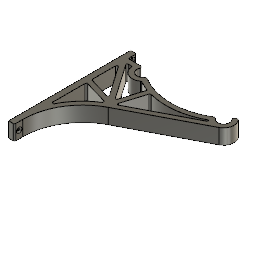
Shelf Bracket Filament (Autodesk Fusion 360 design; units mm, degrees)
Autodesk Fusion 360 part; units mm, degrees
ref_plane "WorkPlane1" through (-87.2, -39.4, 1) normal (0, -1, 0) x (1, 0, 0) in component "Filament Spool v1"
sketch "Sketch1" plane through (0, -39.4, 19) normal (0, -1, 0) x (1, 0, 0) in component "Filament Spool v1"
  line L0 (-70, -19) -> (-70, 13) construction
  line L1 (-81.2, -7.5) -> (-58.8, -7.5) construction
  circle A0 centre (-70, -7.5) radius 12.5 construction
  line L2 (-95.2, -19) -> (95.2, -19) construction
  line L3 (95.2, -19) -> (-95.2, -19) construction
  line L4 (0, -19) -> (0, -95.5696) construction
  line L5 (-70, -7.5) -> (0, -95.5696) construction
  circle A1 centre (0, -95.5696) radius 100
  circle A2 centre (0, -95.5696) radius 16
  circle A3 centre (0, -95.5696) radius 29
  dimension "d141" = 200
  dimension "d142" = 32
  dimension "d143" = 58
  measures "d141" diameter of A1
  measures "d142" diameter of A2
  measures "d143" diameter of A3
extrude "Extrude1" add sketch "Sketch1" against normal blind 31 contours A3 makes body 1 in component "Filament Spool v1"
extrude "Extrude2" add sketch "Sketch1" against normal blind 3 contours A1 bodies 1 in component "Filament Spool v1"
mirror "Mirror1" about plane through (0, -8.4, 19) normal (0, 1, 0) of bodies 1 makes body 2 in component "Filament Spool v1"
ref_plane "WorkPlane1" through (0, -35.4581, -18.5114) normal (0, 0, 1) x (1, 0, 0) in component "Bracket Hollow"
sketch "Shape" plane through (0, -35.4581, -18.5114) normal (0, 0, 1) x (1, 0, 0) in component "Bracket Hollow"
  circle A0 centre (0, 0) radius 100 construction
  circle A1 centre (0, 0) radius 16 construction
  circle A2 centre (-67.4303, -86.3069) radius 9.525 construction
  circle A3 centre (67.4303, -86.3069) radius 9.525 construction
  line L0 (0, 0) -> (0, -254.1299) construction
  line L1 (0, 0) -> (-67.4303, -86.3069) construction
  line L2 (0, 0) -> (67.4303, -86.3069) construction
  arc A4 (-79.6085, -70.7818) -> (83.1792, -66.5492) centre (0, 0) ccw construction
  arc A5 (-72.5254, -78.0234) -> (-58.1603, -89.2466) centre (-67.4303, -86.3069) ccw
  arc A6 (-85.1531, -86.0234) -> (-56.0327, -99.8815) centre (-67.4303, -86.3069) ccw
  arc A7 (58.1603, -89.2466) -> (72.5254, -78.0234) centre (67.4303, -86.3069) ccw
  arc A8 (56.0327, -99.8815) -> (78.2573, -72.2729) centre (67.4303, -86.3069) ccw
  arc A9 (-56.0327, -99.8815) -> (56.0327, -99.8815) centre (0, 0) ccw
  arc A10 (-58.1603, -89.2466) -> (58.1603, -89.2466) centre (0, 0) ccw
  arc A11 (72.5254, -78.0234) -> (78.2573, -72.2729) centre (0, 0) ccw
  line L3 (-85.1531, -86.0234) -> (-100, -86.0234)
  line L4 (-72.5254, -78.0234) -> (-100, -78.0234)
  line L5 (-100, -64.0234) -> (-110, -64.0234)
  line L6 (-110, -64.0234) -> (-110, -268.1299)
  line L7 (-110, -268.1299) -> (-100, -268.1299)
  line L8 (-100, -268.1299) -> (-100, -254.1299)
  line L9 (75.6148, -102.0291) -> (-46.1749, -165.4288)
  arc A12 (-46.1749, -165.4288) -> (-100, -254.1299) centre (0, -254.1299) ccw
  line L10 (67.4303, -86.3069) -> (75.6148, -102.0291) construction
  line L11 (-100, -254.1299) -> (0, -254.1299) construction
  line L12 (0, -254.1299) -> (-49.8689, -158.3328) construction
  line L13 (-49.8689, -158.3328) -> (58.7763, -101.7757)
  line L14 (-100, -64.0234) -> (-100, -268.1299) construction
  arc A13 (-49.8689, -158.3328) -> (-100, -213.3378) centre (0, -254.1299) ccw
  line L15 (-100, -78.0234) -> (-100, -64.0234)
  line L16 (-100, -86.0234) -> (-100, -213.3378)
  line L17 (-100, -86.0234) -> (-49.8689, -158.3328) construction
  line L18 (-95.1327, -86.0234) -> (-46.2923, -156.4709)
  line L19 (-100, -93.044) -> (-53.4023, -160.2566)
  line L20 (-49.8689, -158.3328) -> (0, 0) construction
  line L21 (-49.8689, -158.3328) -> (-100, -143.3378) construction
  line L22 (-51.232, -149.3459) -> (-38.1991, -107.9667)
  line L23 (-30.5687, -110.37) -> (-44.8527, -155.7215)
  line L24 (-54.7631, -161.0439) -> (-100, -147.5129)
  line L25 (-100, -139.1627) -> (-59.6614, -151.2286)
  line L26 (-100, -71.0234) -> (-110, -71.0234) construction
  line L27 (-100, -261.1299) -> (-110, -261.1299) construction
  line L28 (85.1553, -53.7492) -> (85.1553, -190) construction
  dimension "d28" = 19.05
  dimension "d29" = 19.05
  dimension "d33" = 8
  dimension "d36" = 38
  dimension "d37" = 3
  dimension "d38" = 0.2
  dimension "d39" = 8
  dimension "d41" = 0.2
  dimension "d42" = 8
  dimension "d44" = 8
  dimension "d46" = 10
  dimension "d47" = 8
  dimension "d49" = 14
  dimension "d50" = 62.5
  dimension "d51" = 8
  dimension "d52" = 8
  dimension "d53" = 8
  dimension "d54" = 70
  dimension "d60" = 14
  dimension "d61" = 204.8421
  measures "d28" diameter of A2
  measures "d29" diameter of A3
  measures "d33" distance of A9 A10
  measures "d36" angle of L0 L1
  measures "d38" distance of A2 A5
  measures "d39" distance of A5 A6
  measures "d41" distance of A3 A7
  measures "d42" distance of A7 A8
  measures "d47" distance of L3 L4
  measures "d50" angle of L11 L12
  measures "d51" distance of L18 L19
  measures "d52" distance of L24 L25
  measures "d53" distance of L22 L23
  measures "d61" distance of L5 L7
extrude "Extrude1'" add sketch "Shape" along normal mid plane 25.4 separate body contours A5 A7 A8 A10 A11 L4 L5 L6 L7 L8 L9 A12 L15 | L3 L13 A13 L16 L18 L19 | A9 L13 L18 L22 L23 | A13 L16 L19 L24 L25 makes body 3 in component "Bracket Hollow"
fillet "Fillet3" radius 2 18 edges at (-100, -99.4815, -18.5114) (-100, -113.4815, -18.5114) (-95.1327, -121.4815, -18.5114) (-100, -128.5021, -18.5114) (-100, -174.6208, -18.5114) (-100, -182.971, -18.5114) (-100, -248.7959, -18.5114) (-44.8527, -191.1796, -18.5114) (-51.232, -184.804, -18.5114) (-59.6614, -186.6867, -18.5114) (-54.7631, -196.5021, -18.5114) (58.7763, -137.2338, -18.5114) (56.0327, -135.3396, -18.5114) (-30.5687, -145.8281, -18.5114) (-38.1991, -143.4248, -18.5114) (-100, -303.5881, -18.5114) (-56.0327, -135.3396, -18.5114) (-85.1531, -121.4815, -18.5114) on bodies 3 in component "Bracket Hollow"
fillet "Fillet4" radius 3 5 edges at (58.1603, -124.7047, -18.5114) (78.2573, -107.731, -18.5114) (72.5254, -113.4815, -18.5114) (-58.1603, -124.7047, -18.5114) (-72.5254, -113.4815, -18.5114) on bodies 3 in component "Bracket Hollow"
ref_plane "WorkPlane5" through (-110, -201.5348, -18.5114) normal (-1, 0, 0) x (0, -1, 0) in component "Bracket Hollow"
sketch "Screw Holes" plane through (-110, -201.5348, -18.5114) normal (-1, 0, 0) x (0, 1, 0) in component "Bracket Hollow"
  line L0 (-100.0533, -12.7) -> (-100.0533, 12.7) construction
  line L1 (-100.0533, 12.7) -> (-88.0533, 12.7) construction
  line L2 (-88.0533, 12.7) -> (-88.0533, -12.7) construction
  line L3 (-88.0533, -12.7) -> (-100.0533, -12.7) construction
  line L4 (90.0533, -12.7) -> (90.0533, 12.7) construction
  line L5 (90.0533, 12.7) -> (100.0533, 12.7) construction
  line L6 (100.0533, 12.7) -> (100.0533, -12.7) construction
  line L7 (100.0533, -12.7) -> (90.0533, -12.7) construction
  line L8 (95.0533, -12.7) -> (95.0533, 12.7) construction
  line L9 (93.7353, -4.0672) -> (92.4173, -6.35)
  line L10 (92.4173, -6.35) -> (93.7353, -8.6328)
  line L11 (93.7353, -8.6328) -> (96.3712, -8.6328)
  line L12 (96.3712, -8.6328) -> (97.6892, -6.35)
  line L13 (97.6892, -6.35) -> (96.3712, -4.0672)
  line L14 (96.3712, -4.0672) -> (93.7353, -4.0672)
  line L15 (93.7353, 8.6328) -> (92.4173, 6.35)
  line L16 (92.4173, 6.35) -> (93.7353, 4.0672)
  line L17 (93.7353, 4.0672) -> (96.3712, 4.0672)
  line L18 (96.3712, 4.0672) -> (97.6892, 6.35)
  line L19 (97.6892, 6.35) -> (96.3712, 8.6328)
  line L20 (96.3712, 8.6328) -> (93.7353, 8.6328)
  line L21 (-94.0533, -12.7) -> (-94.0533, 12.7) construction
  line L22 (-92.7353, -2.2828) -> (-91.4173, 0)
  line L23 (-91.4173, 0) -> (-92.7353, 2.2828)
  line L24 (-92.7353, 2.2828) -> (-95.3712, 2.2828)
  line L25 (-95.3712, 2.2828) -> (-96.6892, 0)
  line L26 (-96.6892, 0) -> (-95.3712, -2.2828)
  line L27 (-95.3712, -2.2828) -> (-92.7353, -2.2828)
  line L28 (90.0533, 0) -> (100.0533, -12.7) construction
  line L29 (90.0533, 0) -> (100.0533, 12.7) construction
  dimension "d91" = 2.2828
  dimension "d92" = 2.2828
  dimension "d93" = 2.2828
  measures "d91" distance of L14
  measures "d92" distance of L20
  measures "d93" distance of origin L27
extrude "Extrude3" cut sketch "Screw Holes" against normal up to surface (10 mm away) bodies 3 in component "Bracket Hollow"
ref_plane "WorkPlane6" through (-110, -106.4815, -18.5114) normal (0, 1, 0) x (0, 0, -1) in component "Bracket Hollow"
sketch "Screw Bevel Top" plane through (-110, -106.4815, -18.5114) normal (0, 1, 0) x (1, 0, 0) in component "Bracket Hollow"
  line L0 (10, -8.6328) -> (10, -6.35) construction
  line L1 (10, -6.35) -> (10, -4.0672) construction
  line L2 (10, -4.0672) -> (10, -6.35) construction
  line L3 (10, -6.35) -> (10, -8.6328) construction
  line L4 (10, 4.0672) -> (10, 6.35) construction
  line L5 (10, 6.35) -> (10, 8.6328) construction
  line L6 (10, 8.6328) -> (10, 6.35) construction
  line L7 (10, 6.35) -> (10, 4.0672) construction
  line L8 (10, -12.7) -> (10, 12.7) construction
  line L9 (10, 12.7) -> (10, -12.7) construction
  line L10 (0, -6.35) -> (0, -8.6328) construction
  line L11 (0, -8.6328) -> (0, -6.35) construction
  line L12 (0, -6.35) -> (0, -4.0672) construction
  line L13 (0, -4.0672) -> (0, -6.35) construction
  line L14 (0, 6.35) -> (0, 4.0672) construction
  line L15 (0, 4.0672) -> (0, 6.35) construction
  line L16 (0, 6.35) -> (0, 8.6328) construction
  line L17 (0, 8.6328) -> (0, 6.35) construction
  line L18 (0, 0) -> (0, 2.2828) construction
  line L19 (0, 2.2828) -> (0, 0) construction
  line L20 (0, 0) -> (0, -2.2828) construction
  line L21 (0, -2.2828) -> (0, 0) construction
  line L22 (0, 12.7) -> (0, -12.7) construction
  line L23 (0, -12.7) -> (0, 12.7) construction
  line L24 (10, -6.35) -> (0, -6.35) construction
  line L25 (10, 6.35) -> (0, 6.35) construction
  line L26 (10, 1.9336) -> (4.8291, 6.35)
  line L27 (4.8291, 6.35) -> (10, 10.7664) construction
  line L28 (10, -10.7664) -> (4.8291, -6.35)
  line L29 (4.8291, -6.35) -> (10, -1.9336) construction
  line L30 (10, -10.7664) -> (10, -6.35)
  line L31 (10, -6.35) -> (4.8291, -6.35)
  line L32 (10, 1.9336) -> (10, 6.35)
  line L33 (10, 6.35) -> (4.8291, 6.35)
  dimension "d100" = 81
  dimension "d101" = 81
  dimension "d102" = 8.8328
  dimension "d103" = 8.8328
  measures "d100" angle of L26 L27
  measures "d101" angle of L28 L29
revolve "Revolve4" cut sketch "Screw Bevel Top" angle 360 about axis through (-100, -106.4815, -12.1614) along (-1, 0, 0) contours L28 L30 L31 bodies 3 in component "Bracket Hollow"
revolve "Revolve5" cut sketch "Screw Bevel Top" angle 360 about axis through (-100, -106.4815, -24.8614) along (-1, 0, 0) contours L26 L32 L33 bodies 3 in component "Bracket Hollow"
ref_plane "WorkPlane7" through (-110, -295.5881, -18.5114) normal (0, 1, 0) x (0, 0, -1) in component "Bracket Hollow"
sketch "Screw Bevel Bottom" plane through (-110, -295.5881, -18.5114) normal (0, 1, 0) x (1, 0, 0) in component "Bracket Hollow"
  line L0 (10, 2.2828) -> (10, 0) construction
  line L1 (10, 0) -> (10, -2.2828) construction
  line L2 (10, -2.2828) -> (10, 0) construction
  line L3 (10, 0) -> (10, 2.2828) construction
  line L4 (10, -12.7) -> (10, 12.7) construction
  line L5 (10, 12.7) -> (10, -12.7) construction
  line L6 (0, -6.35) -> (0, -8.6328) construction
  line L7 (0, -8.6328) -> (0, -6.35) construction
  line L8 (0, -6.35) -> (0, -4.0672) construction
  line L9 (0, -4.0672) -> (0, -6.35) construction
  line L10 (0, 6.35) -> (0, 4.0672) construction
  line L11 (0, 4.0672) -> (0, 6.35) construction
  line L12 (0, 6.35) -> (0, 8.6328) construction
  line L13 (0, 8.6328) -> (0, 6.35) construction
  line L14 (0, 0) -> (0, 2.2828) construction
  line L15 (0, 2.2828) -> (0, 0) construction
  line L16 (0, 0) -> (0, -2.2828) construction
  line L17 (0, -2.2828) -> (0, 0) construction
  line L18 (0, 12.7) -> (0, -12.7) construction
  line L19 (0, -12.7) -> (0, 12.7) construction
  line L20 (0, 0) -> (10, 0) construction
  line L21 (10, 4.4164) -> (4.8291, 0) construction
  line L22 (4.8291, 0) -> (10, -4.4164)
  line L23 (10, -4.4164) -> (10, 0)
  line L24 (10, 0) -> (4.8291, 0)
  dimension "d107" = 8.8328
  dimension "d108" = 81
  measures "d108" angle of L21 L22
revolve "Revolve6" cut sketch "Screw Bevel Bottom" angle 360 about axis through (-110, -295.5881, -18.5114) along (1, 0, 0) bodies 3 in component "Bracket Hollow"
ref_plane "WorkPlane1" through (0, -35.4581, -18.5114) normal (0, 0, 1) x (1, 0, 0) in component "Bracket Fill"
sketch "Shape (2)" plane through (0, -35.4581, -18.5114) normal (0, 0, 1) x (1, 0, 0) in component "Bracket Fill"
  circle A0 centre (0, 0) radius 100 construction
  circle A1 centre (0, 0) radius 16 construction
  circle A2 centre (-67.4303, -86.3069) radius 9.525 construction
  circle A3 centre (67.4303, -86.3069) radius 9.525 construction
  line L0 (0, 0) -> (0, -254.1299) construction
  line L1 (0, 0) -> (-67.4303, -86.3069) construction
  line L2 (0, 0) -> (67.4303, -86.3069) construction
  arc A4 (-79.6085, -70.7818) -> (83.1792, -66.5492) centre (0, 0) ccw construction
  arc A5 (-72.5254, -78.0234) -> (-58.1603, -89.2466) centre (-67.4303, -86.3069) ccw
  arc A6 (-85.1531, -86.0234) -> (-56.0327, -99.8815) centre (-67.4303, -86.3069) ccw
  arc A7 (58.1603, -89.2466) -> (72.5254, -78.0234) centre (67.4303, -86.3069) ccw
  arc A8 (56.0327, -99.8815) -> (78.2573, -72.2729) centre (67.4303, -86.3069) ccw
  arc A9 (-56.0327, -99.8815) -> (56.0327, -99.8815) centre (0, 0) ccw
  arc A10 (-58.1603, -89.2466) -> (58.1603, -89.2466) centre (0, 0) ccw
  arc A11 (72.5254, -78.0234) -> (78.2573, -72.2729) centre (0, 0) ccw
  line L3 (-85.1531, -86.0234) -> (-100, -86.0234)
  line L4 (-72.5254, -78.0234) -> (-100, -78.0234)
  line L5 (-100, -64.0234) -> (-110, -64.0234)
  line L6 (-110, -64.0234) -> (-110, -268.1299)
  line L7 (-110, -268.1299) -> (-100, -268.1299)
  line L8 (-100, -268.1299) -> (-100, -254.1299)
  line L9 (75.6148, -102.0291) -> (-46.1749, -165.4288)
  arc A12 (-46.1749, -165.4288) -> (-100, -254.1299) centre (0, -254.1299) ccw
  line L10 (67.4303, -86.3069) -> (75.6148, -102.0291) construction
  line L11 (-100, -254.1299) -> (0, -254.1299) construction
  line L12 (0, -254.1299) -> (-49.8689, -158.3328) construction
  line L13 (-49.8689, -158.3328) -> (58.7763, -101.7757)
  line L14 (-100, -64.0234) -> (-100, -268.1299) construction
  arc A13 (-49.8689, -158.3328) -> (-100, -213.3378) centre (0, -254.1299) ccw
  line L15 (-100, -78.0234) -> (-100, -64.0234)
  line L16 (-100, -86.0234) -> (-100, -213.3378)
  line L17 (-100, -86.0234) -> (-49.8689, -158.3328) construction
  line L18 (-95.1327, -86.0234) -> (-46.2923, -156.4709)
  line L19 (-100, -93.044) -> (-53.4023, -160.2566)
  line L20 (-49.8689, -158.3328) -> (0, 0) construction
  line L21 (-49.8689, -158.3328) -> (-100, -143.3378) construction
  line L22 (-51.232, -149.3459) -> (-38.1991, -107.9667)
  line L23 (-30.5687, -110.37) -> (-44.8527, -155.7215)
  line L24 (-54.7631, -161.0439) -> (-100, -147.5129)
  line L25 (-100, -139.1627) -> (-59.6614, -151.2286)
  line L26 (-100, -71.0234) -> (-110, -71.0234) construction
  line L27 (-100, -261.1299) -> (-110, -261.1299) construction
  line L28 (85.1553, -53.7492) -> (85.1553, -190) construction
  dimension "d28_1" = 19.05
  dimension "d29_1" = 19.05
  dimension "d33_1" = 8
  dimension "d36_1" = 38
  dimension "d37_1" = 3
  dimension "d38_1" = 0.2
  dimension "d39_1" = 8
  dimension "d41_1" = 0.2
  dimension "d42_1" = 8
  dimension "d44_1" = 8
  dimension "d46_1" = 10
  dimension "d47_1" = 8
  dimension "d49_1" = 14
  dimension "d50_1" = 62.5
  dimension "d51_1" = 8
  dimension "d52_1" = 8
  dimension "d53_1" = 8
  dimension "d54_1" = 70
  dimension "d60_1" = 14
  dimension "d61_1" = 204.8421
  measures "d28_1" diameter of A2
  measures "d29_1" diameter of A3
  measures "d33_1" distance of A9 A10
  measures "d36_1" angle of L0 L1
  measures "d38_1" distance of A2 A5
  measures "d39_1" distance of A5 A6
  measures "d41_1" distance of A3 A7
  measures "d42_1" distance of A7 A8
  measures "d47_1" distance of L3 L4
  measures "d50_1" angle of L11 L12
  measures "d51_1" distance of L18 L19
  measures "d52_1" distance of L24 L25
  measures "d53_1" distance of L22 L23
  measures "d61_1" distance of L5 L7
extrude "Extrude1''" add sketch "Shape (2)" along normal mid plane 25.4 separate body contours A5 A7 A8 A10 A11 L4 L5 L6 L7 L8 L9 A12 L15 | L3 L13 A13 L16 L18 L19 | A9 L13 L18 L22 L23 | A13 L16 L19 L24 L25 makes body 4 in component "Bracket Fill"
fillet "Fillet3'" radius 2 18 edges at (-100, -99.4815, -18.5114) (-100, -113.4815, -18.5114) (-95.1327, -121.4815, -18.5114) (-100, -128.5021, -18.5114) (-100, -174.6208, -18.5114) (-100, -182.971, -18.5114) (-100, -248.7959, -18.5114) (-44.8527, -191.1796, -18.5114) (-51.232, -184.804, -18.5114) (-59.6614, -186.6867, -18.5114) (-54.7631, -196.5021, -18.5114) (58.7763, -137.2338, -18.5114) (56.0327, -135.3396, -18.5114) (-30.5687, -145.8281, -18.5114) (-38.1991, -143.4248, -18.5114) (-100, -303.5881, -18.5114) (-56.0327, -135.3396, -18.5114) (-85.1531, -121.4815, -18.5114) on bodies 4 in component "Bracket Fill"
fillet "Fillet4'" radius 3 5 edges at (58.1603, -124.7047, -18.5114) (78.2573, -107.731, -18.5114) (72.5254, -113.4815, -18.5114) (-58.1603, -124.7047, -18.5114) (-72.5254, -113.4815, -18.5114) on bodies 4 in component "Bracket Fill"
ref_plane "WorkPlane5" through (-110, -201.5348, -18.5114) normal (-1, 0, 0) x (0, -1, 0) in component "Bracket Fill"
sketch "Screw Holes (2)" plane through (-110, -201.5348, -18.5114) normal (-1, 0, 0) x (0, 1, 0) in component "Bracket Fill"
  line L0 (-100.0533, -12.7) -> (-100.0533, 12.7) construction
  line L1 (-100.0533, 12.7) -> (-88.0533, 12.7) construction
  line L2 (-88.0533, 12.7) -> (-88.0533, -12.7) construction
  line L3 (-88.0533, -12.7) -> (-100.0533, -12.7) construction
  line L4 (90.0533, -12.7) -> (90.0533, 12.7) construction
  line L5 (90.0533, 12.7) -> (100.0533, 12.7) construction
  line L6 (100.0533, 12.7) -> (100.0533, -12.7) construction
  line L7 (100.0533, -12.7) -> (90.0533, -12.7) construction
  line L8 (95.0533, -12.7) -> (95.0533, 12.7) construction
  line L9 (93.7353, -4.0672) -> (92.4173, -6.35)
  line L10 (92.4173, -6.35) -> (93.7353, -8.6328)
  line L11 (93.7353, -8.6328) -> (96.3712, -8.6328)
  line L12 (96.3712, -8.6328) -> (97.6892, -6.35)
  line L13 (97.6892, -6.35) -> (96.3712, -4.0672)
  line L14 (96.3712, -4.0672) -> (93.7353, -4.0672)
  line L15 (93.7353, 8.6328) -> (92.4173, 6.35)
  line L16 (92.4173, 6.35) -> (93.7353, 4.0672)
  line L17 (93.7353, 4.0672) -> (96.3712, 4.0672)
  line L18 (96.3712, 4.0672) -> (97.6892, 6.35)
  line L19 (97.6892, 6.35) -> (96.3712, 8.6328)
  line L20 (96.3712, 8.6328) -> (93.7353, 8.6328)
  line L21 (-94.0533, -12.7) -> (-94.0533, 12.7) construction
  line L22 (-92.7353, -2.2828) -> (-91.4173, 0)
  line L23 (-91.4173, 0) -> (-92.7353, 2.2828)
  line L24 (-92.7353, 2.2828) -> (-95.3712, 2.2828)
  line L25 (-95.3712, 2.2828) -> (-96.6892, 0)
  line L26 (-96.6892, 0) -> (-95.3712, -2.2828)
  line L27 (-95.3712, -2.2828) -> (-92.7353, -2.2828)
  line L28 (90.0533, 0) -> (100.0533, -12.7) construction
  line L29 (90.0533, 0) -> (100.0533, 12.7) construction
  dimension "d91_1" = 2.2828
  dimension "d92_1" = 2.2828
  dimension "d93_1" = 2.2828
  measures "d91_1" distance of L14
  measures "d92_1" distance of L20
  measures "d93_1" distance of origin L27
extrude "Extrude3'" cut sketch "Screw Holes (2)" against normal up to surface (10 mm away) bodies 4 in component "Bracket Fill"
ref_plane "WorkPlane6" through (-110, -106.4815, -18.5114) normal (0, 1, 0) x (0, 0, -1) in component "Bracket Fill"
sketch "Screw Bevel Top (2)" plane through (-110, -106.4815, -18.5114) normal (0, 1, 0) x (1, 0, 0) in component "Bracket Fill"
  line L0 (10, -8.6328) -> (10, -6.35) construction
  line L1 (10, -6.35) -> (10, -4.0672) construction
  line L2 (10, -4.0672) -> (10, -6.35) construction
  line L3 (10, -6.35) -> (10, -8.6328) construction
  line L4 (10, 4.0672) -> (10, 6.35) construction
  line L5 (10, 6.35) -> (10, 8.6328) construction
  line L6 (10, 8.6328) -> (10, 6.35) construction
  line L7 (10, 6.35) -> (10, 4.0672) construction
  line L8 (10, -12.7) -> (10, 12.7) construction
  line L9 (10, 12.7) -> (10, -12.7) construction
  line L10 (0, -6.35) -> (0, -8.6328) construction
  line L11 (0, -8.6328) -> (0, -6.35) construction
  line L12 (0, -6.35) -> (0, -4.0672) construction
  line L13 (0, -4.0672) -> (0, -6.35) construction
  line L14 (0, 6.35) -> (0, 4.0672) construction
  line L15 (0, 4.0672) -> (0, 6.35) construction
  line L16 (0, 6.35) -> (0, 8.6328) construction
  line L17 (0, 8.6328) -> (0, 6.35) construction
  line L18 (0, 0) -> (0, 2.2828) construction
  line L19 (0, 2.2828) -> (0, 0) construction
  line L20 (0, 0) -> (0, -2.2828) construction
  line L21 (0, -2.2828) -> (0, 0) construction
  line L22 (0, 12.7) -> (0, -12.7) construction
  line L23 (0, -12.7) -> (0, 12.7) construction
  line L24 (10, -6.35) -> (0, -6.35) construction
  line L25 (10, 6.35) -> (0, 6.35) construction
  line L26 (10, 1.9336) -> (4.8291, 6.35)
  line L27 (4.8291, 6.35) -> (10, 10.7664) construction
  line L28 (10, -10.7664) -> (4.8291, -6.35)
  line L29 (4.8291, -6.35) -> (10, -1.9336) construction
  line L30 (10, -10.7664) -> (10, -6.35)
  line L31 (10, -6.35) -> (4.8291, -6.35)
  line L32 (10, 1.9336) -> (10, 6.35)
  line L33 (10, 6.35) -> (4.8291, 6.35)
  dimension "d100_1" = 81
  dimension "d101_1" = 81
  dimension "d102_1" = 8.8328
  dimension "d103_1" = 8.8328
  measures "d100_1" angle of L26 L27
  measures "d101_1" angle of L28 L29
revolve "Revolve4'" cut sketch "Screw Bevel Top (2)" angle 360 about axis through (-100, -106.4815, -12.1614) along (-1, 0, 0) contours L28 L30 L31 bodies 4 in component "Bracket Fill"
revolve "Revolve5'" cut sketch "Screw Bevel Top (2)" angle 360 about axis through (-100, -106.4815, -24.8614) along (-1, 0, 0) contours L26 L32 L33 bodies 4 in component "Bracket Fill"
ref_plane "WorkPlane7" through (-110, -295.5881, -18.5114) normal (0, 1, 0) x (0, 0, -1) in component "Bracket Fill"
sketch "Screw Bevel Bottom (2)" plane through (-110, -295.5881, -18.5114) normal (0, 1, 0) x (1, 0, 0) in component "Bracket Fill"
  line L0 (10, 2.2828) -> (10, 0) construction
  line L1 (10, 0) -> (10, -2.2828) construction
  line L2 (10, -2.2828) -> (10, 0) construction
  line L3 (10, 0) -> (10, 2.2828) construction
  line L4 (10, -12.7) -> (10, 12.7) construction
  line L5 (10, 12.7) -> (10, -12.7) construction
  line L6 (0, -6.35) -> (0, -8.6328) construction
  line L7 (0, -8.6328) -> (0, -6.35) construction
  line L8 (0, -6.35) -> (0, -4.0672) construction
  line L9 (0, -4.0672) -> (0, -6.35) construction
  line L10 (0, 6.35) -> (0, 4.0672) construction
  line L11 (0, 4.0672) -> (0, 6.35) construction
  line L12 (0, 6.35) -> (0, 8.6328) construction
  line L13 (0, 8.6328) -> (0, 6.35) construction
  line L14 (0, 0) -> (0, 2.2828) construction
  line L15 (0, 2.2828) -> (0, 0) construction
  line L16 (0, 0) -> (0, -2.2828) construction
  line L17 (0, -2.2828) -> (0, 0) construction
  line L18 (0, 12.7) -> (0, -12.7) construction
  line L19 (0, -12.7) -> (0, 12.7) construction
  line L20 (0, 0) -> (10, 0) construction
  line L21 (10, 4.4164) -> (4.8291, 0) construction
  line L22 (4.8291, 0) -> (10, -4.4164)
  line L23 (10, -4.4164) -> (10, 0)
  line L24 (10, 0) -> (4.8291, 0)
  dimension "d107_1" = 8.8328
  dimension "d108_1" = 81
  measures "d108_1" angle of L21 L22
revolve "Revolve6'" cut sketch "Screw Bevel Bottom (2)" angle 360 about axis through (-110, -295.5881, -18.5114) along (1, 0, 0) bodies 4 in component "Bracket Fill"
extrude "Extrude4" add sketch "Shape (2)" along normal mid plane 1.6 contours A6 A9 L3 L18 L22 | A8 A9 L13 L23 | L16 L19 L25 | A13 L16 L24 bodies 4 in component "Bracket Fill"
chamfer "Chamfer4" distance 0.6 angle 45 58 edges at (56.8878, -137.2057, -17.7114) (7.6252, -163.8614, -17.7114) (-42.7805, -188.7094, -17.7114) (-37.2734, -167.1156, -17.7114) (-30.2059, -146.5064, -17.7114) (14.3515, -149.0804, -17.7114) (55.7714, -135.5337, -17.7114) (55.7714, -135.5337, -19.3114) (14.3515, -149.0804, -19.3114) (-30.2059, -146.5064, -19.3114) (-37.2734, -167.1156, -19.3114) (-42.7805, -188.7094, -19.3114) (7.6252, -163.8614, -19.3114) (56.8878, -137.2057, -19.3114) (-44.3903, -163.0815, -17.7114) (-51.6137, -182.288, -17.7114) (-73.2567, -153.0356, -17.7114) (-93.0844, -122.5539, -17.7114) (-89.1965, -121.4815, -17.7114) (-85.7292, -122.0071, -17.7114) (-74.7863, -137.8915, -17.7114) (-55.973, -135.7334, -17.7114) (-47.557, -139.6421, -17.7114) (-38.8852, -143.7728, -17.7114) (-81.852, -180.0492, -17.7114) (-99.6041, -174.326, -17.7114) (-100, -154.0143, -17.7114) (-98.597, -132.9884, -17.7114) (-79.6352, -157.8764, -17.7114) (-62.9388, -184.309, -17.7114) (-80.1342, -217.1829, -17.7114) (-98.4671, -241.5728, -17.7114) (-100, -212.6424, -17.7114) (-99.1945, -184.0527, -17.7114) (-78.2318, -189.4822, -17.7114) (-57.6297, -196.8587, -17.7114) (-80.1342, -217.1829, -19.3114) (-57.6297, -196.8587, -19.3114) (-78.2318, -189.4822, -19.3114) (-99.1945, -184.0527, -19.3114) (-100, -212.6424, -19.3114) (-98.4671, -241.5728, -19.3114) (-81.852, -180.0492, -19.3114) (-62.9388, -184.309, -19.3114) (-79.6352, -157.8764, -19.3114) (-98.597, -132.9884, -19.3114) (-100, -154.0143, -19.3114) (-99.6041, -174.326, -19.3114) (-44.3903, -163.0815, -19.3114) (-38.8852, -143.7728, -19.3114) (-47.557, -139.6421, -19.3114) (-55.973, -135.7334, -19.3114) (-74.7863, -137.8915, -19.3114) (-85.7292, -122.0071, -19.3114) (-89.1965, -121.4815, -19.3114) (-93.0844, -122.5539, -19.3114) (-73.2567, -153.0356, -19.3114) (-51.6137, -182.288, -19.3114) on bodies 4 in component "Bracket Fill"
component "Filament Spool v1" placed x (1, 0, 0) y (0, 0, 1) z (0, -1, 0) at (0, -112.0277, -41.1114)
component "Bracket Hollow" placed x (1, 0, 0) y (0, 1, 0) z (0, 0, 1) at (0, 0, 0)
component "Bracket Fill" placed x (1, 0, 0) y (0, 1, 0) z (0, 0, 1) at (0, 0, 0)
equation "rod_diameter = 0.75 in"
equation "rod_clearance = 0.4 mm"
equation "rod_hole = rod_diameter + rod_clearance"
equation "screw_shank = 0.164 in"
equation "screw_clearance = 0.4 mm"
equation "screw_hole = screw_shank + screw_clearance"
equation "screw_head = 0.332 in"
equation "screw_head_hole = screw_head + screw_clearance"
equation "screw_head_angle = 81 deg"
equation "d28 = rod_diameter"
equation "d29 = rod_diameter"
equation "frame_thickness = 8 mm"
equation "d33 = frame_thickness"
equation "d38 = rod_clearance / 2"
equation "d39 = frame_thickness"
equation "d41 = rod_clearance / 2"
equation "d42 = frame_thickness"
equation "d44 = frame_thickness"
equation "back_thickness = 10 mm"
equation "d46 = back_thickness"
equation "d47 = frame_thickness"
equation "d51 = frame_thickness"
equation "d52 = frame_thickness"
equation "d53 = frame_thickness"
equation "d91 = screw_hole / 2"
equation "d92 = screw_hole / 2"
equation "d93 = screw_hole / 2"
equation "d100 = screw_head_angle"
equation "d101 = screw_head_angle"
equation "d102 = screw_head_hole"
equation "d103 = screw_head_hole"
equation "d107 = screw_head_hole"
equation "d108 = screw_head_angle"
equation "d28_1 = rod_diameter"
equation "d29_1 = rod_diameter"
equation "d33_1 = frame_thickness"
equation "d38_1 = rod_clearance / 2"
equation "d39_1 = frame_thickness"
equation "d41_1 = rod_clearance / 2"
equation "d42_1 = frame_thickness"
equation "d44_1 = frame_thickness"
equation "d46_1 = back_thickness"
equation "d47_1 = frame_thickness"
equation "d51_1 = frame_thickness"
equation "d52_1 = frame_thickness"
equation "d53_1 = frame_thickness"
equation "d91_1 = screw_hole / 2"
equation "d92_1 = screw_hole / 2"
equation "d93_1 = screw_hole / 2"
equation "d100_1 = screw_head_angle"
equation "d101_1 = screw_head_angle"
equation "d102_1 = screw_head_hole"
equation "d103_1 = screw_head_hole"
equation "d107_1 = screw_head_hole"
equation "d108_1 = screw_head_angle"
